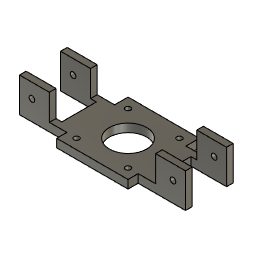
z_motor_mount (Autodesk Fusion 360 design; units mm, degrees)
Autodesk Fusion 360 part; units mm, degrees
sketch "Sketch1" plane through (0, 0, 0) normal (0, 0, 1) x (1, 0, 0)
  line L0 (0, 0) -> (58, 0)
  line L1 (58, 0) -> (58, 20)
  line L2 (58, 20) -> (0, 20)
  line L3 (0, 20) -> (0, 0)
  dimension "d1" = 58
  dimension "d2" = 20
  constraint horizontal L0
  constraint vertical L1
  constraint horizontal L2
  constraint vertical L3
  constraint coincident L0.start L3.end
  measures "d1" distance of L0.start L0.end
  measures "d2" distance of L0.start L2.end
extrude "Extrude1" add sketch "Sketch1" along normal blind 5 makes body 1
sketch "Sketch2" plane through (0, 0, 5) normal (0, 0, 1) x (-1, 0, 0)
  line L0 (0, -20) -> (0, 0)
  line L1 (0, 0) -> (-58, 0)
  line L2 (-58, 0) -> (-58, -20)
  line L3 (-58, -20) -> (0, -20)
  line L4 (-7.5, -32.5) -> (-50.5, -32.5)
  line L5 (-50.5, -32.5) -> (-50.5, 10.5)
  line L6 (-50.5, 10.5) -> (-7.5, 10.5)
  line L7 (-7.5, 10.5) -> (-7.5, -32.5)
  dimension "d5" = 43
  dimension "d6" = 43
  dimension "d7" = 7.5
  dimension "d8" = 12.5
  dimension "d9" = 11
  constraint horizontal L4
  constraint vertical L5
  constraint horizontal L6
  constraint vertical L7
  measures "d5" distance of L4.start L4.end
  measures "d6" distance of L4.start L6.end
  measures "d7" distance of L0 L7
  measures "d8" distance of L3 L4
extrude "Extrude2" add sketch "Sketch2" against normal blind 5 contours L3 L4 L5 L7 | L1 L5 L6 L7 bodies 1
sketch "Sketch3" plane through (0, 0, 0) normal (-1, 0, 0) x (0, -1, 0)
  line L0 (-20, 0) -> (0, 0)
  line L1 (0, 0) -> (0, 5)
  line L2 (0, 5) -> (-20, 5)
  line L3 (-20, 5) -> (-20, 0)
  line L4 (-20, 5) -> (0, 5)
  line L5 (0, 5) -> (0, 35)
  line L6 (0, 35) -> (-20, 35)
  line L7 (-20, 35) -> (-20, 5)
  dimension "d12" = 30
  dimension "d13" = 20
  constraint horizontal L4
  constraint vertical L5
  constraint horizontal L6
  constraint vertical L7
  constraint coincident L2.end L3.start
  measures "d12" distance of L2.end L6.end
  measures "d13" distance of L2.end L1.end
extrude "Extrude3" add sketch "Sketch3" against normal blind 5 contours L2 L4 L5 L6 L7 bodies 1
sketch "Sketch4" plane through (58, 0, 0) normal (1, 0, 0) x (0, 1, 0)
  line L0 (0, 0) -> (20, 0)
  line L1 (20, 0) -> (20, 5)
  line L2 (20, 5) -> (0, 5)
  line L3 (0, 5) -> (0, 0)
  line L4 (0, 5) -> (20, 5)
  line L5 (20, 5) -> (20, 35)
  line L6 (20, 35) -> (0, 35)
  line L7 (0, 35) -> (0, 5)
  dimension "d16" = 30
  dimension "d17" = 20
  constraint horizontal L4
  constraint vertical L5
  constraint horizontal L6
  constraint vertical L7
  constraint coincident L2.end L3.start
  measures "d16" distance of L2.end L6.end
  measures "d17" distance of L2.end L1.end
extrude "Extrude4" add sketch "Sketch4" against normal blind 5 contours L2 L4 L5 L6 L7 bodies 1
sketch "Sketch5" plane through (58, 0, 0) normal (1, 0, 0) x (0, 1, 0)
  line L0 (0, 0) -> (20, 0)
  line L1 (20, 0) -> (20, 35)
  line L2 (20, 35) -> (0, 35)
  line L3 (0, 35) -> (0, 0)
  point P0 (9.722, 25)
  point P1 (9.722, 13)
  dimension "d20" = 10
  dimension "d21" = 12
  measures "d20" distance of L2 P0
  measures "d21" distance of P0 P1
hole "Hole1" at (58, 9.722, 25) at (58, 9.722, 13) direction (-1, 0, 0) diameter 3.2 depth 300 tip angle 118 bodies 1
sketch "Sketch6" plane through (0, 0, 0) normal (0, 0, -1) x (1, 0, 0)
  line L0 (0, 0) -> (0, -20)
  line L1 (0, -20) -> (7.5, -20)
  line L2 (7.5, -20) -> (7.5, -32.5)
  line L3 (7.5, -32.5) -> (50.5, -32.5)
  line L4 (50.5, -32.5) -> (50.5, -20)
  line L5 (50.5, -20) -> (58, -20)
  line L6 (58, -20) -> (58, 0)
  line L7 (58, 0) -> (50.5, 0)
  line L8 (50.5, 0) -> (50.5, 10.5)
  line L9 (50.5, 10.5) -> (7.5, 10.5)
  line L10 (7.5, 10.5) -> (7.5, 0)
  line L11 (7.5, 0) -> (0, 0)
  point P0 (13.5, 4.5)
  point P1 (44.5, 4.5)
  point P2 (44.5, -26.5)
  point P3 (13.5, -26.5)
  dimension "d25" = 31
  dimension "d26" = 31
  dimension "d27" = 31
  dimension "d28" = 31
  dimension "d29" = 6
  dimension "d30" = 7
  dimension "d31" = 6
  constraint horizontal P0 P1
  constraint vertical P1 P2
  measures "d25" distance of P0 P1
  measures "d26" vertical distance of P0 P3
  measures "d27" vertical distance of P1 P2
  measures "d28" distance of P2 P3
  measures "d29" distance of L9 P0
  measures "d31" distance of L8 P1
hole "Hole2" at (13.5, -4.5, 0) at (44.5, -4.5, 0) at (44.5, 26.5, 0) at (13.5, 26.5, 0) direction (0, 0, 1) diameter 3.2 depth 300 tip angle 118 bodies 1
sketch "Sketch7" plane through (0, 0, 0) normal (0, 0, -1) x (1, 0, 0)
  circle A0 centre (44.5, -26.5) radius 1.6
  circle A1 centre (13.5, 4.5) radius 1.6
  circle A2 centre (44.5, 4.5) radius 1.6
  circle A3 centre (13.5, -26.5) radius 1.6
  line L0 (0, 0) -> (0, -20)
  line L1 (0, -20) -> (7.5, -20)
  line L2 (7.5, -20) -> (7.5, -32.5)
  line L3 (7.5, -32.5) -> (50.5, -32.5)
  line L4 (50.5, -32.5) -> (50.5, -20)
  line L5 (50.5, -20) -> (58, -20)
  line L6 (58, -20) -> (58, 0)
  line L7 (58, 0) -> (50.5, 0)
  line L8 (50.5, 0) -> (50.5, 10.5)
  line L9 (50.5, 10.5) -> (7.5, 10.5)
  line L10 (7.5, 10.5) -> (7.5, 0)
  line L11 (7.5, 0) -> (0, 0)
  point P0 (29, -11)
  dimension "d35" = 29
  dimension "d36" = 29
  dimension "d37" = 21.5
  dimension "d38" = 20
  measures "d35" distance of L0 P0
  measures "d36" distance of L6 P0
  measures "d37" distance of L9 P0
hole "Hole3" at (29, 11, 0) direction (0, 0, 1) diameter 22.5 depth 300 tip angle 118 bodies 1
copy_body "Body->Comp1" bodies 1 removing the originals makes body 2 in component "z_motor_mount"
extrude "Extrude1'" cut 1 faces at (53, 17.094, 21.548) along direction (1, 0, 0) blind 3 on bodies 2 bodies 2 in component "z_motor_mount"
extrude "Extrude2'" add 1 faces at (58, 9.9073, 3.8) along direction (1, 0, 0) blind 3 on bodies 2 bodies 2 in component "z_motor_mount"
extrude "Extrude3'" cut 1 faces at (5, 17.094, 21.548) along direction (-1, 0, 0) blind 3 on bodies 2 bodies 2 in component "z_motor_mount"
extrude "Extrude4'" add 1 faces at (0, 9.9073, 3.8) along direction (-1, 0, 0) blind 3 on bodies 2 bodies 2 in component "z_motor_mount"
extrude "Extrude5" add 1 faces at (-3, 9.9073, 3.8) along direction (-1, 0, 0) blind 20.1 on bodies 2 bodies 2 in component "z_motor_mount"
extrude "Extrude6" cut 1 faces at (2, 17.094, 21.548) along direction (-1, 0, 0) blind 20.1 on bodies 2 bodies 2 in component "z_motor_mount"
extrude "Extrude7" add 1 faces at (61, 9.9073, 3.8) along direction (1, 0, 0) blind 20.1 on bodies 2 bodies 2 in component "z_motor_mount"
extrude "Extrude8" cut 1 faces at (56, 17.094, 21.548) along direction (1, 0, 0) blind 20.1 on bodies 2 bodies 2 in component "z_motor_mount"
sketch "Sketch8" plane through (0, 0, 35) normal (0, 0, 1) x (-1, 0, 0)
  line L0 (18.1, 0) -> (18.1, -20)
  line L1 (18.1, -20) -> (23.1, -20)
  line L2 (23.1, -20) -> (23.1, 0)
  line L3 (23.1, 0) -> (18.1, 0)
extrude "Extrude9" cut sketch "Sketch8" against normal up to surface (30 mm away) bodies 2 in component "z_motor_mount"
extrude "Extrude10" cut 1 faces at (77.7667, 13.3333, 35) along direction (0, 0, -1) up to surface (30 mm away) on bodies 2 bodies 2 in component "z_motor_mount"
sketch "Sketch9" plane through (0, 0, 0) normal (0, -1, 0) x (1, 0, 0)
  line L0 (81.1, 5) -> (50.5, 5)
  line L1 (50.5, 5) -> (50.5, 0)
  line L2 (50.5, 0) -> (81.1, 0)
  line L3 (81.1, 0) -> (81.1, 5)
  line L4 (-1, 0) -> (-21, 0)
  line L5 (-21, 0) -> (-21, 30)
  line L6 (-21, 30) -> (-1, 30)
  line L7 (-1, 30) -> (-1, 0)
  line L8 (59, 0) -> (79, 0)
  line L9 (79, 0) -> (79, 30)
  line L10 (79, 30) -> (59, 30)
  line L11 (59, 30) -> (59, 0)
  line L12 (-23.1, 5) -> (-23.1, 0)
  point P0 (50.5, 5)
  point P1 (7.5, 5)
  dimension "d62" = 20
  dimension "d63" = 30
  dimension "d64" = 20
  dimension "d65" = 30
  dimension "d66" = 100
  dimension "d67" = 60
  dimension "d71" = 8.5
  dimension "d72" = 7
  constraint horizontal L4
  constraint vertical L5
  constraint horizontal L6
  constraint vertical L7
  constraint horizontal L8
  constraint vertical L9
  constraint horizontal L10
  constraint vertical L11
  constraint coincident L2 L8.start
  measures "d62" distance of L4.start L4.end
  measures "d63" distance of L4.start L6.end
  measures "d64" distance of L8.start L8.end
  measures "d65" distance of L8.start L10.end
  measures "d66" distance of L5 L9
  measures "d67" distance of L7 L11
  measures "d71" distance of L11 P0
extrude "Extrude11" add sketch "Sketch9" along normal blind 4 contours L0 L2 L8 L9 L11 | L0 L9 L10 L11 | L4 L5 L6 L7 bodies 2 in component "z_motor_mount"
sketch "Sketch10" plane through (0, -4, 0) normal (0, -1, 0) x (1, 0, 0)
  line L0 (-1, 30) -> (-21, 30)
  line L1 (-21, 30) -> (-21, 0)
  line L2 (-21, 0) -> (-1, 0)
  line L3 (-1, 0) -> (-1, 30)
  line L4 (59, 30) -> (59, 0)
  line L5 (59, 0) -> (79, 0)
  point P0 (-11, 15)
  point P1 (69, 15)
  dimension "d75" = 15
  dimension "d76" = 10
  dimension "d77" = 10
  dimension "d78" = 15
  measures "d75" distance of L2 P0
  measures "d76" distance of L3 P0
  measures "d77" distance of P1 L4
  measures "d78" distance of P1 L5
hole "Hole1'" at (-11, -4, 15) at (69, -4, 15) direction (0, 1, 0) diameter 3.4 depth 40 tip angle 118 bodies 2 in component "z_motor_mount"
extrude "Extrude12" cut 2 faces at (-14.3333, -2.6667, 30) (72.3333, -2.6667, 30) along direction (0, 0, -1) blind 3.4 on bodies 2 bodies 2 in component "z_motor_mount"
extrude "Extrude13" add 2 faces at (-14.3333, -2.6667, 26.6) (72.3333, -2.6667, 26.6) along direction (0, 0, 1) blind 0.1 on bodies 2 bodies 2 in component "z_motor_mount"
ref_plane "WorkPlane1" through (0, 11, 0) normal (0, 1, 0) x (0, 0, 1)
sketch "Sketch11" plane through (0, 20, 0) normal (0, 1, 0) x (-1, 0, 0)
  line L0 (-50.5, 5) -> (-81.1, 5)
  line L1 (-81.1, 5) -> (-81.1, 0)
  line L2 (-81.1, 0) -> (-50.5, 0)
  line L3 (-50.5, 0) -> (-50.5, 5)
sketch "Sketch12" plane through (0, 20, 0) normal (0, 1, 0) x (-1, 0, 0)
  line L0 (-78.9615, 4.9735) -> (-58.9615, 4.9735)
  line L1 (-58.9615, 4.9735) -> (-58.9615, 26.584)
  line L2 (-58.9615, 26.584) -> (-78.9615, 26.584)
  line L3 (-78.9615, 26.584) -> (-78.9615, 4.9735)
  line L4 (1.0522, 4.9247) -> (21.0522, 4.9247)
  line L5 (21.0522, 4.9247) -> (21.0522, 26.6893)
  line L6 (21.0522, 26.6893) -> (1.0522, 26.6893)
  line L7 (1.0522, 26.6893) -> (1.0522, 4.9247)
  dimension "d87" = 20
  dimension "d88" = 20
  constraint horizontal L0
  constraint vertical L1
  constraint horizontal L2
  constraint vertical L3
  constraint horizontal L4
  constraint vertical L5
  constraint horizontal L6
  constraint vertical L7
  measures "d87" distance of L0.start L0.end
  measures "d88" distance of L4.start L4.end
extrude "Extrude14" add sketch "Sketch12" along normal blind 4 bodies 2 in component "z_motor_mount"
extrude "Extrude15" add 1 faces at (72.2949, 22.6667, 4.9735) along direction (0, 0, -1) up to surface (4.9735 mm away) on bodies 2 bodies 2 in component "z_motor_mount"
extrude "Extrude16" add 1 faces at (-7.7189, 21.3333, 4.9247) along direction (0, 0, -1) up to surface (4.9247 mm away) on bodies 2 bodies 2 in component "z_motor_mount"
extrude "Extrude17" add 1 faces at (58.9615, 22.6667, 10.528) along direction (-1, 0, 0) up to surface (8.4615 mm away) on bodies 2 bodies 2 in component "z_motor_mount"
extrude "Extrude18" cut 1 faces at (50.5, 21.3333, 19.3893) along direction (1, 0, 0) up to surface (8.5 mm away) on bodies 2 bodies 2 in component "z_motor_mount"
extrude "Extrude19" add 1 faces at (59, -2.6667, 10.5667) along direction (-1, 0, 0) up to surface (8.5 mm away) on bodies 2 bodies 2 in component "z_motor_mount"
extrude "Extrude20" cut 1 faces at (50.5, -1.3333, 19.4667) along direction (1, 0, 0) up to surface (8.5 mm away) on bodies 2 bodies 2 in component "z_motor_mount"
extrude "Extrude21" cut 1 faces at (81.1, 6.6667, 3.3333) along direction (-1, 0, 0) up to surface (30.6 mm away) on bodies 2 bodies 2 in component "z_motor_mount"
extrude "Extrude22" add 1 faces at (50.5, 6.6667, 3.3333) along direction (1, 0, 0) blind 7 on bodies 2 bodies 2 in component "z_motor_mount"
extrude "Extrude23" add 1 faces at (-1.0522, 22.6667, 10.5631) along direction (1, 0, 0) up to surface (8.5522 mm away) on bodies 2 bodies 2 in component "z_motor_mount"
extrude "Extrude24" cut 1 faces at (7.5, 21.3333, 19.4595) along direction (-1, 0, 0) up to surface (8.5 mm away) on bodies 2 bodies 2 in component "z_motor_mount"
extrude "Extrude25" add 1 faces at (-1, -2.6667, 10.5667) along direction (1, 0, 0) up to surface (8.5 mm away) on bodies 2 bodies 2 in component "z_motor_mount"
extrude "Extrude26" cut 1 faces at (7.5, -1.3333, 19.4667) along direction (-1, 0, 0) up to surface (8.5 mm away) on bodies 2 bodies 2 in component "z_motor_mount"
extrude "Extrude27" cut 1 faces at (-23.1, 13.3333, 3.3333) along direction (1, 0, 0) up to surface (30.6 mm away) on bodies 2 bodies 2 in component "z_motor_mount"
extrude "Extrude28" add 1 faces at (7.5, 13.3333, 3.3333) along direction (-1, 0, 0) blind 7 on bodies 2 bodies 2 in component "z_motor_mount"
sketch "Sketch13" plane through (0, 24, 0) normal (0, 1, 0) x (-1, 0, 0)
  line L0 (-59, 5) -> (-59, 26.584)
  line L1 (-59, 26.584) -> (-78.9615, 26.584)
  line L2 (-78.9615, 26.584) -> (-78.9615, 0)
  line L3 (-78.9615, 0) -> (-50.5, 0)
  line L4 (-50.5, 0) -> (-50.5, 5)
  line L5 (-50.5, 5) -> (-59, 5)
  line L6 (21.0522, 0) -> (-7.5, 0)
  line L7 (1, 26.6893) -> (1, 5)
  point P0 (-69, 15)
  point P1 (11, 15)
  dimension "d119" = 15
  dimension "d120" = 15
  dimension "d121" = 10
  dimension "d122" = 10
  measures "d119" distance of L3 P0
  measures "d120" distance of P1 L6
  measures "d121" distance of P1 L7
  measures "d122" distance of L0 P0
hole "Hole2'" at (69, 24, 15) at (-11, 24, 15) direction (0, -1, 0) diameter 3.4 depth 40 tip angle 118 bodies 2 in component "z_motor_mount"
extrude "Extrude29" cut 2 faces at (-11.0174, 20, 6.1) (68.9872, 20, 6.1) along direction (0, 1, 0) blind 0.2 on bodies 2 bodies 2 in component "z_motor_mount"
extrude "Extrude30" add 2 faces at (68.9872, 24, 6.1) (-11.0174, 24, 6.1) along direction (0, 1, 0) blind 0.2 on bodies 2 bodies 2 in component "z_motor_mount"
extrude "Extrude31" cut 2 faces at (69, 0, 6.1) (-11, 0, 6.1) along direction (0, -1, 0) blind 0.2 on bodies 2 bodies 2 in component "z_motor_mount"
extrude "Extrude32" add 1 faces at (-11, -4, 6.1) along direction (0, -1, 0) blind 0.2 on bodies 2 bodies 2 in component "z_motor_mount"
move_face "MoveFace1" to x (1, 0, 0) y (0, 1, 0) z (0, 0, 1) at (-0.0224, 0, -2.9999) 4 faces at (-11.1693, -1.5333, 13.3084) (-10.8307, 21.5333, 16.6916) (68.3397, 22.8667, 16.5665) (67.9073, -1.4667, 13.6977) on bodies 2 in component "z_motor_mount"
extrude "Extrude33" cut 1 faces at (72.3077, 21.5333, 26.584) along direction (0, 0, -1) blind 3 on bodies 2 bodies 2 in component "z_motor_mount"
extrude "Extrude34" cut 1 faces at (72.3333, -1.4667, 26.7) along direction (0, 0, -1) blind 3 on bodies 2 bodies 2 in component "z_motor_mount"
extrude "Extrude35" cut 1 faces at (-14.3333, -2.8667, 26.7) along direction (0, 0, -1) blind 3 on bodies 2 bodies 2 in component "z_motor_mount"
extrude "Extrude36" cut 1 faces at (-14.3682, 21.5333, 26.6893) along direction (0, 0, -1) blind 3 on bodies 2 bodies 2 in component "z_motor_mount"
move_face "MoveFace2" to x (1, 0, 0) y (0, 1, 0) z (0, 0, 1) at (-2.5, 0, -0.0099) 1 faces at (-10.8531, 21.5333, 13.6916) on bodies 2 in component "z_motor_mount"
extrude "Extrude37" cut 1 faces at (-1, 21.5333, 11.2298) along direction (-1, 0, 0) blind 2 on bodies 2 bodies 2 in component "z_motor_mount"
extrude "Extrude38" cut 1 faces at (-1, -1.5333, 11.2333) along direction (-1, 0, 0) blind 2 on bodies 2 bodies 2 in component "z_motor_mount"
move_face "MoveFace3" to x (1, 0, 0) y (0, 1, 0) z (0, 0, 1) at (-2.4999, 0, 0.0212) 1 faces at (-11.1916, -1.5333, 10.3085) on bodies 2 in component "z_motor_mount"
extrude "Extrude39" cut 2 faces at (59, -1.4667, 11.2333) (59, 21.5333, 11.1947) along direction (1, 0, 0) blind 2 on bodies 2 bodies 2 in component "z_motor_mount"
move_face "MoveFace4" to x (0.998879, 0, -0.047338) y (0, 1, 0) z (0.047338, 0, 0.998879) at (2.0085, 0, 3.2165) 1 faces at (69.638, 21.5333, 13.5666) on bodies 2 in component "z_motor_mount"
move_face "MoveFace5" to x (1, 0, 0) y (0, 1, 0) z (0, 0, 1) at (2.5081, 0, -0.0298) 1 faces at (67.8849, -1.4667, 13.3024) on bodies 2 in component "z_motor_mount"
extrude "Extrude40" cut 2 faces at (73, -1.4667, 23.7) (-15, -1.5333, 23.7) along direction (0, 0, -1) blind 3 on bodies 2 bodies 2 in component "z_motor_mount"
extrude "Extrude41" cut 1 faces at (72.9744, 21.5333, 23.584) along direction (0, 0, -1) blind 3 on bodies 2 bodies 2 in component "z_motor_mount"
extrude "Extrude42" cut 1 faces at (-15.0348, 21.5333, 23.6893) along direction (0, 0, -1) blind 3 on bodies 2 bodies 2 in component "z_motor_mount"
extrude "Extrude43" cut 1 faces at (63.9298, 20.2, 12.5763) along direction (0, 1, 0) blind 0.2 on bodies 2 bodies 2 in component "z_motor_mount"
extrude "Extrude44" add 2 faces at (63.9298, 24.2, 12.5763) (-5.9424, 24.2, 12.6022) along direction (0, 1, 0) blind 0.2 on bodies 2 bodies 2 in component "z_motor_mount"
extrude "Extrude45" cut 2 faces at (63.9302, -0.2, 12.5991) (-5.9423, -0.2, 12.6161) along direction (0, -1, 0) blind 0.2 on bodies 2 bodies 2 in component "z_motor_mount"
extrude "Extrude46" add 1 faces at (63.9302, -4, 12.5991) along direction (0, -1, 0) blind 0.2 on bodies 2 bodies 2 in component "z_motor_mount"
extrude "Extrude47" add 1 faces at (-5.9423, -4.2, 12.6161) along direction (0, -1, 0) blind 0.2 on bodies 2 bodies 2 in component "z_motor_mount"
extrude "Extrude48" add 1 faces at (63.9302, -4.2, 12.5991) along direction (0, -1, 0) blind 0.2 on bodies 2 bodies 2 in component "z_motor_mount"
extrude "Extrude49" cut 1 faces at (-5.9424, 20.2, 12.6022) along direction (0, 1, 0) blind 0.2 on bodies 2 bodies 2 in component "z_motor_mount"
component "z_motor_mount" placed x (1, 0, 0) y (0, 1, 0) z (0, 0, 1) at (0, 0, 0)
equation "d7 = ( ( 58 - 43 ) / 2 ) * 1 mm"
